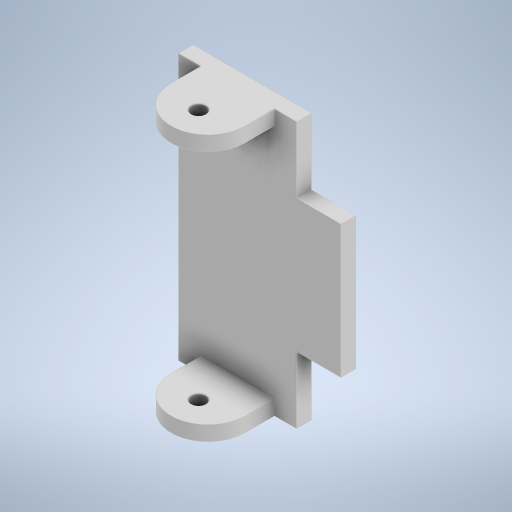
# Autodesk Inventor part: wheel_braket
Saved by Autodesk Inventor 2023 (Build 270158000, 158)
## iProperties
Created: 2024-02-05
Part Number: wheel_braket
Material: PBT 플라스틱
Document SubType Name: Modeling
Designer: ps737
Density: 1.31 g/cm^3
Appearance: 암회색
Author: ps737
Autodesk Inventor part; units mm, degrees
ref_plane "YZ Plane" through (0, 0, 0) normal (1, 0, 0) x (0, 1, 0)
ref_plane "XZ Plane" through (0, 0, 0) normal (0, 1, 0) x (-1, 0, 0)
ref_plane "XY Plane" through (0, 0, 0) normal (0, 0, 1) x (1, 0, 0)
ref_plane "작업 평면9" through (0, 0, -30) normal (0, 0, 1) x (1, 0, 0)
sketch "스케치7" plane through (0, 0, -30) normal (0, 0, 1) x (1, 0, 0)
  line L0 (0, 0) -> (-40, 0)
  line L1 (-40, 0) -> (-40, 90)
  line L2 (-40, 90) -> (40, 90)
  line L3 (40, 90) -> (40, 45)
  line L4 (40, 45) -> (70, 45)
  line L5 (70, 45) -> (70, 0)
  line L6 (-88.2304, 0) -> (94.9618, 0) construction
  line L7 (-40, 0) -> (-40, -90)
  line L8 (-40, -90) -> (40, -90)
  line L9 (40, -90) -> (40, -45)
  line L10 (40, -45) -> (70, -45)
  line L11 (70, -45) -> (70, 0)
  circle A0 centre (0, 47.0427) radius 7.5 projected
  circle A1 centre (0, -47.0427) radius 7.5 projected
  circle A2 centre (0, 47.0427) radius 7.5
  circle A3 centre (0, -47.0427) radius 7.5
  dimension "d27" = 40
  dimension "d28" = 90
  dimension "d29" = 80
  dimension "d30" = 30
  dimension "d51" = 90
  dimension "d52" = 45
  dimension "d53" = 24.9618
  dimension "d54" = 45
  dimension "d55" = 158.2304
  constraints: 24 end point, 4 perpendicular, 4 symmetric about line, 3 horizontal, 2 centre point, 2 coincident, 2 concentric
  measures "d27" distance of L0.start L0.end
  measures "d28" distance of L0.end L1.end
  measures "d29" distance of L1.end L2.end
  measures "d30" distance of L3.end L4.end
  measures "d51" distance between parallel lines of L10 L4
  measures "d52" distance between parallel lines of L4 L2
  measures "d53" distance from line of L6.end L5
  measures "d54" distance from line of L5.end L4
  measures "d55" distance from line of L6.start L5
extrude "돌출6" add sketch "스케치7" along normal blind 10 contours L1 L2 L3 L4 L5 L11 L10 L9 L8 L7 | A0 | A1
ref_plane "작업 평면12" through (0, 0, -20) normal (0, 0, 1) x (1, 0, 0)
sketch "스케치8" plane through (0, 0, -20) normal (0, 0, 1) x (1, 0, 0)
  line L0 (-40, 90) -> (40, 90) projected
  line L1 (0, 90) -> (25, 90)
  line L2 (25, 90) -> (-25, 90)
  line L3 (-25, 90) -> (-25, 80)
  line L4 (-25, 80) -> (25, 80)
  line L5 (25, 80) -> (25, 90)
  line L6 (40, -90) -> (-40, -90) projected
  line L7 (-25, -90) -> (25, -90)
  line L8 (25, -90) -> (25, -80)
  line L9 (25, -80) -> (-25, -80)
  line L10 (-25, -80) -> (-25, -90)
  point P0 (0, 0)
  dimension "d33" = 25
  dimension "d34" = 50
  dimension "d35" = 10
  dimension "d36" = 10
  constraints: 18 end point, 4 point on line, 3 perpendicular, 2 vertical, 1 midpoint, 1 parallel
  measures "d33" distance of L1.start L1.end
  measures "d34" distance of L1.end L2.end
  measures "d35" distance of L2.end L3.end
  measures "d36" distance of L7.end L8.end
extrude "돌출7" add sketch "스케치8" along normal blind 20
ref_plane "작업 평면5" through (-25, -80, -20) normal (0, 1, 0) x (1, 0, 0)
sketch "스케치9" plane through (-25, -80, -20) normal (0, 1, 0) x (1, 0, 0)
  line L0 (50, -20) -> (0, -20) projected
  circle A0 centre (25, -20) radius 25
  line L1 (0, -20) -> (50, -20) projected
  constraints: 1 coincident, 3 other
ref_plane "작업 평면4" through (-25, 80, -20) normal (0, -1, 0) x (1, 0, 0)
sketch "스케치10" plane through (-25, 80, -20) normal (0, -1, 0) x (1, 0, 0)
  line L0 (0, 20) -> (50, 20) projected
  circle A0 centre (25, 20) radius 25
  constraints: 1 coincident, 3 other
extrude "돌출8" add sketch "스케치10" against normal blind 10 contours A0 L0 picked at (24.1509, 35.7929)
extrude "돌출9" add sketch "스케치9" against normal blind 10 contours A0 L0 picked at (23.041, -32.1453)
ref_plane "작업 평면6" through (-25, 80, -20) normal (0, -1, 0) x (1, 0, 0)
sketch "스케치11" plane through (-25, 80, -20) normal (0, -1, 0) x (1, 0, 0)
  line L0 (-245, 26.4038) -> (295, 26.4038) projected
  circle A0 centre (25, 26.4038) radius 5
  point P0 (25, 20)
  dimension "d43" = 10
  constraints: 1 centre point, 1 midpoint
  measures "d43" diameter of A0
ref_plane "작업 평면7" through (-25, -80, -20) normal (0, 1, 0) x (1, 0, 0)
sketch "스케치12" plane through (-25, -80, -20) normal (0, 1, 0) x (1, 0, 0)
  line L0 (295, -26.4038) -> (-245, -26.4038) projected
  circle A0 centre (25, -26.4038) radius 5
  point P0 (25, -20)
  dimension "d44" = 10
  constraints: 1 centre point, 1 midpoint
  measures "d44" diameter of A0
extrude "돌출10" cut sketch "스케치12" against normal blind 10
extrude "돌출11" cut sketch "스케치11" against normal blind 10
ref_plane "작업 평면8" through (0, -47.0427, -30) normal (0, 0, -1) x (-1, 0, 0)
sketch "스케치13" plane through (0, -47.0427, -30) normal (0, 0, -1) x (-1, 0, 0)
  circle A0 centre (0, 0) radius 7.5
  circle A1 centre (0, 94.0854) radius 7.5 projected
  circle A2 centre (0, 94.0854) radius 7.5
  point P0 (0, 47.0427)
  constraints: 2 centre point, 1 coincident
extrude "돌출12" add sketch "스케치13" along normal blind 30
